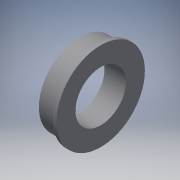
# Autodesk Inventor part: F6804
Saved by Autodesk Inventor 2019.4 (Build 234330000, 330)
## iProperties
Created: 2019-12-12
Part Number: F6804
Material: Generic
Document SubType Name: Modeling
Designer: Mark
Density: 1 g/cm^3
Appearance: Default
Author: Mark
Autodesk Inventor part; units mm, degrees
ref_plane "YZ Plane" through (0, 0, 0) normal (1, 0, 0) x (0, 1, 0)
ref_plane "XZ Plane" through (0, 0, 0) normal (0, 1, 0) x (-1, 0, 0)
ref_plane "XY Plane" through (0, 0, 0) normal (0, 0, 1) x (1, 0, 0)
sketch "Sketch1" plane through (0, 0, 0) normal (1, 0, 0) x (0, 1, 0)
  circle A0 centre (0, 0) radius 10
  circle A1 centre (0, 0) radius 16
  dimension "d0" = 20
  dimension "d1" = 32
  constraints: 2 centre point, 1 coincident, 1 concentric
  measures "d0" diameter of A0
  measures "d1" diameter of A1
extrude "Extrusion1" add sketch "Sketch1" along normal blind 7
sketch "Sketch2" plane through (7, 0, 0) normal (1, 0, 0) x (0, 0, -1)
  circle A0 centre (0, 0) radius 10
  circle A1 centre (0, 0) radius 17.5
  dimension "d4" = 20
  dimension "d5" = 35
  constraints: 2 centre point, 2 coincident
  measures "d4" diameter of A0
  measures "d5" diameter of A1
extrude "Extrusion2" add sketch "Sketch2" along normal blind 1.5
body "Solid1"
